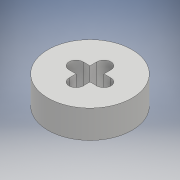
# Autodesk Inventor part: SpacerAxel1
Saved by Autodesk Inventor 2017 (Build 210142000, 142)
## iProperties
Created: 2016-10-28
Part Number: SpacerAxel1
Material: Generic
Document SubType Name: Modeling
Designer: JJ
Density: 1 g/cm^3
Appearance: Default
Author: JJ
Autodesk Inventor part; units mm, degrees
ref_plane "YZ Plane" through (0, 0, 0) normal (1, 0, 0) x (0, 1, 0)
ref_plane "XZ Plane" through (0, 0, 0) normal (0, 1, 0) x (-1, 0, 0)
ref_plane "XY Plane" through (0, 0, 0) normal (0, 0, 1) x (1, 0, 0)
sketch "Sketch1" plane through (0, 0, 0) normal (0, 0, 1) x (1, 0, 0)
  circle A0 centre (0, 0) radius 15
  dimension "d0" = 30
  constraints: 1 centre point, 1 coincident
  measures "d0" diameter of A0
extrude "Extrusion1" add sketch "Sketch1" along normal blind 10
sketch "Sketch2" plane through (0, 0, 10) normal (0, 0, 1) x (1, 0, 0)
  circle A0 centre (0, 0) radius 15 projected
  line L0 (0, -5) -> (0, 5) construction
  line L1 (2.5, -5) -> (2.5, 5)
  line L2 (-2.5, 5) -> (-2.5, -5)
  arc A1 (-2.5, -5) -> (2.5, -5) centre (0, -5) ccw
  arc A2 (2.5, 5) -> (-2.5, 5) centre (0, 5) ccw
  line L3 (5, 0) -> (-5, 0) construction
  line L4 (5, 2.5) -> (-5, 2.5)
  line L5 (-5, -2.5) -> (5, -2.5)
  arc A3 (5, -2.5) -> (5, 2.5) centre (5, 0) ccw
  arc A4 (-5, 2.5) -> (-5, -2.5) centre (-5, 0) ccw
  dimension "d3" = 5
  dimension "d4" = 5
  dimension "d5" = 5
  dimension "d6" = 5
  constraints: 16 end point, 8 point on circle, 8 tangent, 4 centre point, 2 midpoint, 2 parallel, 1 horizontal, 1 vertical
  measures "d3" distance of A0.centre L0.end
  measures "d4" diameter of A2
  measures "d5" distance of A0.centre L3.end
  measures "d6" diameter of A4
extrude "Extrusion2" cut sketch "Sketch2" against normal blind 10 contours A1 L2 L5 L1 | L5 L2 L4 L1 | L1 L4 A3 L5 | L4 L2 A2 L1 | L5 A4 L4 L2
body "Solid1"
